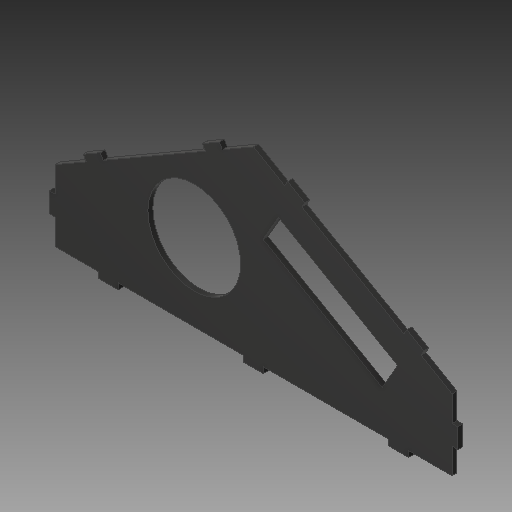
# Autodesk Inventor part: BA19
Saved by Autodesk Inventor 2017 (Build 210142000, 142)
## iProperties
Created: 2019-06-03
Part Number: BA19
Material: Polyethylene, High Density
Document SubType Name: Modeling
Designer: Dell
Density: 0.952 g/cm^3
Appearance: Smooth - Black
Mass: 486.674 g
Surface Area: 1727.68 cm^2
Volume: 511.212 cm^3
Author: Dell
Autodesk Inventor part; units mm, degrees
ref_plane "YZ Plane" through (0, 0, 0) normal (1, 0, 0) x (0, 1, 0)
ref_plane "XZ Plane" through (0, 0, 0) normal (0, 1, 0) x (-1, 0, 0)
ref_plane "XY Plane" through (0, 0, 0) normal (0, 0, 1) x (1, 0, 0)
sketch "Sketch1" plane through (0, 0, 0) normal (0, 0, 1) x (1, 0, 0)
  line L0 (0, 303.5592) -> (262.89, 151.7796) construction
  line L1 (262.89, 151.7796) -> (262.89, -151.7796) construction
  line L2 (262.89, -151.7796) -> (0, -303.5592) construction
  line L3 (0, -303.5592) -> (-262.89, -151.7796) construction
  line L4 (-262.89, -151.7796) -> (-262.89, 151.7796) construction
  line L5 (-262.89, 151.7796) -> (0, 303.5592) construction
  line L6 (0, 296.2269) -> (256.54, 148.1134)
  line L7 (256.54, 148.1134) -> (256.54, -148.1134)
  line L8 (256.54, -148.1134) -> (0, -296.2269)
  line L9 (0, -296.2269) -> (-256.54, -148.1134)
  line L10 (-256.54, -148.1134) -> (-256.54, 148.1134)
  line L11 (-256.54, 148.1134) -> (0, 296.2269)
  line L12 (-256.54, 56.5296) -> (256.54, 56.5296)
  line L13 (256.54, 148.1134) -> (256.54, 56.5296)
  line L14 (-256.54, 56.5296) -> (-256.54, 148.1134)
  point P0 (0, 0)
  point P1 (0, 0)
  point P2 (-256.54, 0)
  dimension "d0" = 525.78
  dimension "d1" = 6.35
  dimension "d2" = 95.25
  constraints: 30 end point, 2 collinear, 2 point on line, 1 coincident, 1 horizontal alignment, 1 midpoint, 1 perpendicular, 18 other
  measures "d0" distance between parallel lines of L1 L4
  measures "d1" distance between parallel lines of L5 L11
  measures "d2" distance from line of L4.end L12
extrude "Extrusion1" add sketch "Sketch1" along normal blind 6.35 contours L6 L7 L12 L10 L11
sketch "Sketch2" plane through (0, 0, 6.35) normal (0, 0, 1) x (1, 0, 0)
  line L0 (-256.54, 56.5296) -> (256.54, 56.5296) projected
  line L1 (-200.2, 56.5296) -> (-174.8, 56.5296)
  line L2 (-174.8, 56.5296) -> (-174.8, 48.9096)
  line L3 (-174.8, 48.9096) -> (-200.2, 48.9096)
  line L4 (-200.2, 48.9096) -> (-200.2, 56.5296)
  line L5 (12.7, 56.5296) -> (-12.7, 56.5296)
  line L6 (-12.7, 56.5296) -> (-12.7, 48.9096)
  line L7 (-12.7, 48.9096) -> (12.7, 48.9096)
  line L8 (12.7, 48.9096) -> (12.7, 56.5296)
  line L9 (174.8, 56.5296) -> (200.2, 56.5296)
  line L10 (200.2, 56.5296) -> (200.2, 48.9096)
  line L11 (200.2, 48.9096) -> (174.8, 48.9096)
  line L12 (174.8, 48.9096) -> (174.8, 56.5296)
  line L13 (256.54, 56.5296) -> (256.54, 148.1134) projected
  line L14 (-256.54, 148.1134) -> (-256.54, 56.5296) projected
  line L15 (-256.54, 115.0215) -> (-264.16, 115.0215)
  line L16 (-264.16, 115.0215) -> (-264.16, 89.6215)
  line L17 (-264.16, 89.6215) -> (-256.54, 89.6215)
  line L18 (-256.54, 89.6215) -> (-256.54, 115.0215)
  line L19 (256.54, 115.0215) -> (264.16, 115.0215)
  line L20 (264.16, 115.0215) -> (264.16, 89.6215)
  line L21 (264.16, 89.6215) -> (256.54, 89.6215)
  line L22 (256.54, 89.6215) -> (256.54, 115.0215)
  line L23 (256.54, 148.1134) -> (0, 296.2269) projected
  line L24 (40.2818, 272.9702) -> (44.0918, 279.5693)
  line L25 (44.0918, 279.5693) -> (66.0889, 266.8693)
  line L26 (66.0889, 266.8693) -> (62.2789, 260.2702)
  line L27 (62.2789, 260.2702) -> (40.2818, 272.9702)
  line L28 (216.2582, 171.3702) -> (220.0682, 177.9693)
  line L29 (220.0682, 177.9693) -> (198.0711, 190.6693)
  line L30 (198.0711, 190.6693) -> (194.2611, 184.0702)
  line L31 (194.2611, 184.0702) -> (216.2582, 171.3702)
  line L32 (66.0889, 266.8693) -> (198.0711, 190.6693) construction
  line L33 (132.08, 228.7693) -> (128.27, 222.1702)
  line L34 (0, 296.2269) -> (0, 336.1275)
  line L35 (-40.2818, 272.9702) -> (-44.0918, 279.5693)
  line L36 (-44.0918, 279.5693) -> (-66.0889, 266.8693)
  line L37 (-66.0889, 266.8693) -> (-62.2789, 260.2702)
  line L38 (-62.2789, 260.2702) -> (-40.2818, 272.9702)
  line L39 (-216.2582, 171.3702) -> (-220.0682, 177.9693)
  line L40 (-220.0682, 177.9693) -> (-198.0711, 190.6693)
  line L41 (-198.0711, 190.6693) -> (-194.2611, 184.0702)
  line L42 (-194.2611, 184.0702) -> (-216.2582, 171.3702)
  line L43 (-66.0889, 266.8693) -> (-198.0711, 190.6693) construction
  line L44 (-132.08, 228.7693) -> (-128.27, 222.1702)
  line L45 (-187.5, 48.9096) -> (187.5, 48.9096) construction
  point P0 (0, 0)
  point P1 (-256.54, 102.3215)
  point P2 (256.54, 102.3215)
  point P3 (0, 56.5296)
  point P4 (0, 48.9096)
  point P5 (0, 56.5296)
  dimension "d5" = 25.4
  dimension "d6" = 7.62
  dimension "d9" = 25.4
  dimension "d10" = 25.4
  dimension "d15" = 7.62
  dimension "d16" = 25.4
  dimension "d17" = 7.62
  dimension "d18" = 25.4
  dimension "d19" = 7.62
  dimension "d20" = 152.4
  dimension "d21" = 25.4
  dimension "d22" = 25.4
  dimension "d30" = 375
  constraints: 84 end point, 14 parallel, 12 midpoint, 10 perpendicular, 10 point on line, 10 symmetric about line, 5 horizontal, 2 horizontal alignment, 1 vertical, 1 vertical alignment
  measures "d5" distance of L2.end L3.end
  measures "d6" distance of L1.end L2.end
  measures "d9" distance of L6.end L7.end
  measures "d10" distance of L10.end L11.end
  measures "d15" distance of L17.end L16.end
  measures "d16" distance of L15.end L16.end
  measures "d17" distance of L20.end L21.end
  measures "d18" distance of L19.end L20.end
  measures "d19" distance of L24.start L24.end
  measures "d20" distance of L25.end L29.end
  measures "d21" distance of L24.end L25.end
  measures "d22" distance of L28.end L29.end
  measures "d30" distance of L45.start L45.end
extrude "Extrusion2" add sketch "Sketch2" against normal blind 6.35
sketch "Sketch3" plane through (0, 0, 6.35) normal (0, 0, 1) x (1, 0, 0)
  line L0 (32.2303, 233.6246) -> (186.2097, 144.7246)
  line L1 (186.2097, 144.7246) -> (166.2097, 110.0836)
  line L2 (166.2097, 110.0836) -> (12.2303, 198.9836)
  line L3 (12.2303, 198.9836) -> (32.2303, 233.6246)
  line L4 (256.54, 148.1134) -> (0, 296.2269) projected
  line L5 (128.27, 222.1702) -> (109.22, 189.1746)
  point P0 (0, 0)
  point P1 (194.2611, 184.0702)
  point P2 (62.2789, 260.2702)
  dimension "d25" = 177.8
  dimension "d26" = 38.1
  dimension "d27" = 40
  constraints: 10 end point, 3 parallel, 2 midpoint, 2 perpendicular
  measures "d25" distance of L1.end L2.end
  measures "d26" distance between parallel lines of L4 L0
  measures "d27" distance of L2.end L0.start
extrude "Extrusion3" cut sketch "Sketch3" against normal through all
sketch "Sketch4" plane through (0, 0, 6.35) normal (0, 0, 1) x (1, 0, 0)
  circle A0 centre (-76.54, 156.5296) radius 60
  line L0 (-174.8, 56.5296) -> (-12.7, 56.5296) projected
  line L1 (-256.54, 148.1134) -> (-256.54, 115.0215) projected
  point P0 (0, 0)
  dimension "d31" = 120
  dimension "d32" = 100
  dimension "d33" = 180
  constraints: 1 centre point
  measures "d31" diameter of A0
  measures "d32" distance from line of L0 A0.centre
  measures "d33" distance from line of L1 A0.centre
extrude "Extrusion4" cut sketch "Sketch4" against normal through all
equation "\"d1\" = Panel_Thickness"
equation "\"d3\" = Panel_Thickness"
equation "\"d6\" = Panel_Thickness + Fit_Tolerance"
equation "\"d15\" = Panel_Thickness + Fit_Tolerance"
equation "\"d17\" = Panel_Thickness + Fit_Tolerance"
equation "\"d19\" = Panel_Thickness + Fit_Tolerance"
equation "\"d23\" = Panel_Thickness"
equation "\"d28\" = Panel_Thickness"
equation "\"d34\" = Panel_Thickness"
equation "\"Panel_Thickness\" = 6.35"
equation "\"Fit_Tolerance\" = 1.27"
equation "\"Tool_Dia\" = 6.35"
body "Solid1"
